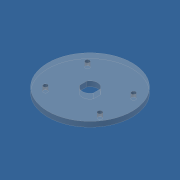
# Autodesk Inventor part: S1702_couverclehaut
Saved by Autodesk Inventor 2015 SP2 (Build 190223200, 223)
## iProperties
Created: 2017-10-31
Part Number: S1702_couverclehaut
Project: S1702_Circuit_Course
Material: Plastique PMMA
Description: Couvercle Haut
Document SubType Name: Modeling
Designer: Benoit.CURCHOD2
Authority: Ø50x3
Density: 1.188 g/cm^3
Appearance: Transparent - Clair
Mass: 6.45604 g
Surface Area: 44.316 cm^2
Volume: 5.43438 cm^3
Material number: ---
Author: Benoit.CURCHOD2
Autodesk Inventor part; units mm, degrees
ref_plane "Plan YZ" through (0, 0, 0) normal (1, 0, 0) x (0, 1, 0)
ref_plane "Plan XZ" through (0, 0, 0) normal (0, 1, 0) x (-1, 0, 0)
ref_plane "Plan XY" through (0, 0, 0) normal (0, 0, 1) x (1, 0, 0)
sketch "Esquisse1" plane through (0, 0, 0) normal (0, 0, 1) x (1, 0, 0)
  circle A0 centre (0, 0) radius 25
  dimension "d0" = 50
  constraints: 1 centre point, 1 coincident
  measures "d0" diameter of A0
extrude "Extrusion1" add sketch "Esquisse1" along normal blind 3
sketch "Esquisse7" plane through (0, 0, 3) normal (0, 0, 1) x (1, 0, 0)
  line L0 (-35, 0) -> (35, 0) construction
  line L1 (0, -35) -> (0, 35) construction
  line L2 (-4.05, -2.0736) -> (-4.05, 2.0736)
  line L3 (4.05, -2.0736) -> (4.05, 2.0736)
  arc A0 (-4.05, -2.0736) -> (4.05, -2.0736) centre (0, 0) ccw
  arc A1 (4.05, 2.0736) -> (-4.05, 2.0736) centre (0, 0) ccw
  dimension "d31" = 8.1
  dimension "d32" = 4.55
  constraints: 4 end point, 4 point on circle, 2 centre point, 2 midpoint, 1 parallel, 1 vertical, 2 other
  measures "d31" distance between parallel lines of L3 L2
  measures "d32" radius of A0
extrude "Extrusion3" cut sketch "Esquisse7" against normal through all
sketch "Esquisse8" plane through (0, 0, 3) normal (0, 0, 1) x (1, 0, 0)
  circle A0 centre (0, 0) radius 18.8 construction
  line L0 (-35, 0) -> (35, 0) construction
  point P0 (-14.0424, 12.5)
  point P1 (-14.0424, -12.5)
  point P2 (15.9198, 10)
  point P3 (15.9198, -10)
  dimension "d16" = 37.6
  dimension "d25" = 25
  dimension "d26" = 20
  constraints: 4 point on circle, 2 symmetric about line, 1 centre point, 1 coincident
  measures "d16" diameter of A0
  measures "d25" distance of A0.end A0.start
  measures "d26" distance of point (15.92, -10) point (15.92, 10)
hole "Perçage1" at (-14.0424, -12.5, 3) at (-14.0424, 12.5, 3) at (15.9198, 10, 3) at (15.9198, -10, 3) direction (0, 0, -1) diameter 2.459 depth 8.5 tip angle 118 thread size "M3x0.5" class "6H" standard "ISO M"
